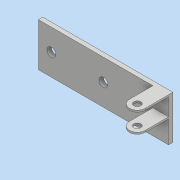
# Autodesk Inventor part: Giá đỡ ròng rọc 2
Saved by Autodesk Inventor 2018 (Build 220112000, 112)
## iProperties
Created: 2020-08-11
Part Number: Giá đỡ ròng rọc 2
Material: Generic
Document SubType Name: Modeling
Designer: ASUS
Density: 1 g/cm^3
Appearance: Default
Author: ASUS
Autodesk Inventor part; units mm, degrees
ref_plane "YZ Plane" through (0, 0, 0) normal (1, 0, 0) x (0, 1, 0)
ref_plane "XZ Plane" through (0, 0, 0) normal (0, 1, 0) x (-1, 0, 0)
ref_plane "XY Plane" through (0, 0, 0) normal (0, 0, 1) x (1, 0, 0)
sketch "Sketch1" plane through (0, 0, 0) normal (0, 1, 0) x (-1, 0, 0)
  line L0 (0, 0) -> (150, 0)
  line L1 (150, 0) -> (150, -50)
  line L2 (150, -50) -> (0, -50)
  line L3 (0, -50) -> (0, 0)
  dimension "d0" = 150
  dimension "d1" = 50
  constraints: 8 end point, 2 parallel, 1 horizontal, 1 perpendicular
  measures "d0" distance of L1.end L2.end
  measures "d1" distance of L0.end L1.end
extrude "Extrusion1" add sketch "Sketch1" along normal blind 5
sketch "Sketch2" plane through (0, 5, 0) normal (0, 1, 0) x (1, 0, 0)
  circle A0 centre (-135, 25) radius 5
  line L0 (-150, 0) -> (0, 0) projected
  line L1 (-150, 50) -> (-150, 0) projected
  circle A1 centre (-75, 25) radius 5
  dimension "d4" = 10
  dimension "d5" = 25
  dimension "d6" = 15
  dimension "d7" = 10
  dimension "d8" = 25
  dimension "d9" = 60
  constraints: 2 centre point
  measures "d4" diameter of A0
  measures "d5" distance from line of L0 A0.centre
  measures "d6" distance from line of L1 A0.centre
  measures "d7" diameter of A1
  measures "d8" distance from line of L0 A1.centre
  measures "d9" distance of A0.centre A1.centre
extrude "Extrusion2" cut sketch "Sketch2" against normal blind 5
sketch "Sketch4" plane through (0, 0, 0) normal (0, -1, 0) x (1, 0, 0)
  line L0 (0, 0) -> (0, -50) projected
  line L1 (0, 0) -> (-18, 0)
  line L2 (-18, 0) -> (-18, -2)
  line L3 (-18, -2) -> (0, -2)
  line L4 (0, -2) -> (0, 0)
  line L5 (0, -22) -> (-18, -22)
  line L6 (-18, -22) -> (-18, -24)
  line L7 (-18, -24) -> (0, -24)
  line L8 (0, -24) -> (0, -22)
  dimension "d17" = 18
  dimension "d18" = 2
  dimension "d19" = 18
  dimension "d20" = 2
  dimension "d21" = 20
  constraints: 16 end point, 4 parallel, 2 horizontal, 2 perpendicular, 1 point on line
  measures "d17" distance of L3.end L2.end
  measures "d18" distance of L2.end L1.end
  measures "d19" distance of L7.end L6.end
  measures "d20" distance of L6.end L5.end
  measures "d21" distance between parallel lines of L3 L5
extrude "Extrusion4" add sketch "Sketch4" along normal blind 36
sketch "Sketch5" plane through (-150, 5, 0) normal (0, 0, 1) x (1, 0, 0)
  circle A0 centre (141, -32) radius 9
  line L0 (150, -41) -> (150, 0) projected
  line L1 (150, -41) -> (132, -41) projected
  line L2 (150, -32) -> (150, -41)
  line L3 (132, -41) -> (132, -32)
  line L4 (132, -5) -> (132, -41) projected
  line L5 (132, -41) -> (150, -41)
  circle A1 centre (141, -32) radius 4
  point P0 (150, -5)
  dimension "d24" = 18
  dimension "d25" = 9
  dimension "d26" = 9
  dimension "d27" = 8
  constraints: 6 end point, 2 centre point, 2 point on circle, 2 point on line, 1 coincident, 1 collinear, 1 perpendicular
  measures "d24" diameter of A0
  measures "d25" distance from line of L0 A0.centre
  measures "d26" distance from line of L1 A0.centre
  measures "d27" diameter of A1
extrude "Extrusion5" cut sketch "Sketch5" against normal blind 36 contours L0 L1 A0 | A0 L1 L3 | A1
body "Solid1"
